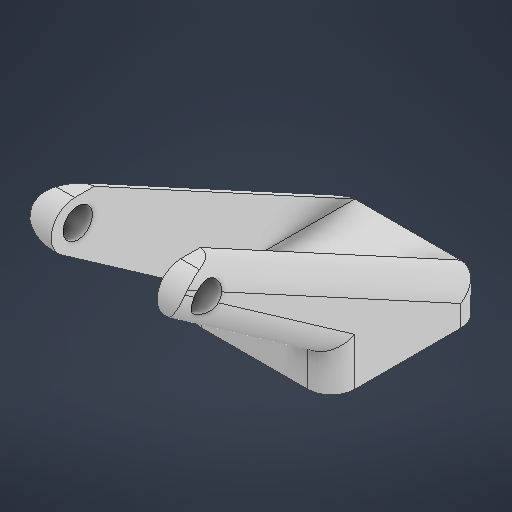
# Autodesk Inventor part: PodstawkaKola
Saved by Autodesk Inventor 2026 (Build 300175000, 175)
## iProperties
Created: 2025-04-29
Part Number: PodstawkaKola
Material: Generic
Document SubType Name: Modeling
Designer: isan
Density: 1 g/cm^3
Appearance: Default
Author: isan
Autodesk Inventor part; units mm, degrees
ref_plane "YZ Plane" through (0, 0, 0) normal (1, 0, 0) x (0, 1, 0)
ref_plane "XZ Plane" through (0, 0, 0) normal (0, 1, 0) x (-1, 0, 0)
ref_plane "XY Plane" through (0, 0, 0) normal (0, 0, 1) x (1, 0, 0)
sketch "Sketch1" plane through (0, 0, 0) normal (0, 0, 1) x (1, 0, 0)
  line L0 (6.5, 6.5) -> (-6.5, 6.5)
  line L1 (-6.5, 6.5) -> (-6.5, -6.5)
  line L2 (-6.5, -6.5) -> (6.5, -6.5)
  line L3 (6.5, -6.5) -> (6.5, 6.5)
  line L4 (6.5, 6.5) -> (-6.5, -6.5) construction
  line L5 (-6.5, 6.5) -> (6.5, -6.5) construction
  point P0 (0, 0)
  point P1 (0, 0)
  dimension "d35" = 13
  dimension "d36" = 13
  constraints: 12 end point, 2 parallel, 1 coincident, 1 horizontal, 1 midpoint, 1 perpendicular
  measures "d35" distance of L1.end L2.end
  measures "d36" distance of L0.end L1.end
extrude "Extrusion1" add sketch "Sketch1" along normal blind 3
sketch "Sketch2" plane through (0, 0, 0) normal (0, 0, -1) x (-1, 0, 0)
  line L0 (-6.5, 1) -> (6.5, 1)
  line L1 (6.5, 1) -> (6.5, -1)
  line L2 (6.5, -1) -> (-6.5, -1)
  line L3 (-6.5, -1) -> (-6.5, 1)
  line L4 (-6.5, 1) -> (6.5, -1) construction
  line L5 (6.5, 1) -> (-6.5, -1) construction
  circle A0 centre (0, 0) radius 4.9
  point P0 (4.7969, 1)
  point P1 (-4.7969, 1)
  point P2 (-4.7969, -1)
  point P3 (4.7969, -1)
  dimension "d3" = 2
  dimension "d4" = 13
  dimension "d57" = 9.8
  constraints: 12 end point, 2 midpoint, 2 parallel, 1 centre point, 1 coincident, 1 horizontal, 1 perpendicular
  measures "d3" distance of L0.end L1.end
  measures "d4" distance of L1.end L2.end
  measures "d57" diameter of A0
extrude "Extrusion2" cut sketch "Sketch2" against normal blind 1.1 contours L0 A0 L2
sketch "Sketch22" plane through (6.5, -6.5, 0) normal (1, 0, 0) x (0, 0, -1)
  line L0 (0, 13) -> (-3, 13) projected
  line L1 (-3, 13) -> (-3, 0) projected
  line L2 (-3, 13) -> (-3, 0)
  line L3 (-3, 0) -> (-15, -17.1378)
  line L4 (-15, -17.1378) -> (-15, -9.1378)
  line L5 (-15, -9.1378) -> (-3, 13)
  line L6 (0, 0) -> (0, 13) projected
  point P0 (0, 6.5)
  point P1 (0, 6.5)
  dimension "d131" = 145
  dimension "d132" = 8
  dimension "d133" = 15
  constraints: 8 end point, 1 midpoint, 1 parallel, 1 vertical
  measures "d131" angle of L3 L1
  measures "d132" distance of L3.end L4.end
  measures "d133" horizontal distance of L3.end point (0, 6.5)
extrude "Extrusion20" add sketch "Sketch22" against normal blind 2
sketch "Sketch24" plane through (6.5, -6.5, 0) normal (1, 0, 0) x (0, 0, -1)
  circle A0 centre (-13, -10.5382) radius 1.25
  line L0 (0, 0) -> (0, 13) projected
  line L1 (-3, 13) -> (-15, -9.1378) projected
  line L2 (-15, -17.1378) -> (-3, 0) projected
  line L3 (-14.7588, -9.3067) -> (-11.2412, -11.7697) construction
  line L4 (-15, -17.1378) -> (-15, -9.1378) projected
  point P0 (0, 6.5)
  point P1 (0, 6.5)
  dimension "d141" = 2.5
  dimension "d142" = 13
  dimension "d149" = 90
  constraints: 2 end point, 2 midpoint, 2 point on line, 1 centre point, 1 coincident
  measures "d141" diameter of A0
  measures "d142" horizontal distance of point (0, 6.5) A0.centre
  measures "d149" angle of L2 L3
extrude "Extrusion22" cut sketch "Sketch24" against normal blind 2
mirror "Mirror2" about plane through (0, 0, 0) normal (1, 0, 0) of "Extrusion20", "Extrusion22"
fillet "Fillet6" radius 2 10 edges at (-5.5, -23.6378, 15) (5.5, -23.6378, 15) (-6.5, -4.5689, 9) (6.5, -4.5689, 9) (-6.5, 6.5, 1.5) (-6.5, -15.0689, 9) (-6.5, -6.5, 1.5) (6.5, -15.0689, 9) (6.5, -6.5, 1.5) (6.5, 6.5, 1.5)
body "Solid1"
